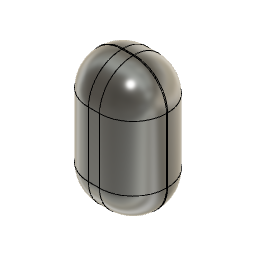
pill v1 (Autodesk Fusion 360 design; units mm, degrees)
Autodesk Fusion 360 part; units mm, degrees
sketch "Sketch1" plane through (0, 0, 0) normal (0, 1, 0) x (1, 0, 0)
  line L0 (0, 0) -> (7, 0)
  line L1 (7, 0) -> (7, -11.8)
  line L2 (7, -11.8) -> (0, -11.8)
  line L3 (0, -11.8) -> (0, 0)
  dimension "d1" = 7
  dimension "d2" = 11.8
  constraint horizontal L0
  constraint vertical L1
  constraint horizontal L2
  constraint vertical L3
  constraint coincident L0.start L3.end
  measures "d1" distance of L1.end L2.end
  measures "d2" distance of L0.end L1.end
extrude "Extrude1" add sketch "Sketch1" along normal blind 6.1
fillet "Fillet1" radius 3 12 edges at (7, 3.05, 11.8) (3.5, 0, 11.8) (0, 3.05, 11.8) (3.5, 6.1, 11.8) (7, 0, 5.9) (7, 3.05, 0) (3.5, 0, 0) (7, 6.1, 5.9) (0, 0, 5.9) (3.5, 6.1, 0) (0, 6.1, 5.9) (0, 3.05, 0)
